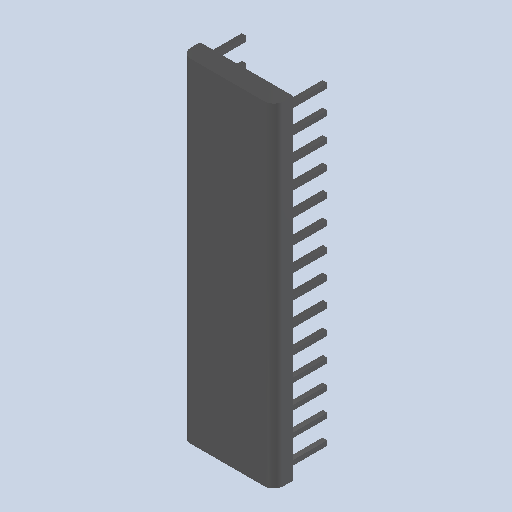
# Autodesk Inventor part: ATMEGA328P-PV
Saved by Autodesk Inventor 2022 (Build 260153000, 153)
## iProperties
Created: 2017-06-03
Part Number: ATMEGA328P-PV
Material: Rubber
Document SubType Name: Modeling
Designer: L.Đ.P
Density: 0.93 g/cm^3
Appearance: Rubber - Black - Version 1.1
Mass: 0.646794 g
Surface Area: 10.546 cm^2
Volume: 0.695478 cm^3
Author: L.Đ.P
Autodesk Inventor part; units mm, degrees
ref_plane "YZ Plane" through (0, 0, 0) normal (1, 0, 0) x (0, 1, 0)
ref_plane "XZ Plane" through (0, 0, 0) normal (0, 1, 0) x (-1, 0, 0)
ref_plane "XY Plane" through (0, 0, 0) normal (0, 0, 1) x (1, 0, 0)
sketch "Sketch1" plane through (0, 0, 0) normal (0, 0, 1) x (1, 0, 0)
  line L0 (0.625, 15.75) -> (0.625, 16.75) projected
  line L1 (0.625, 16.75) -> (-0.625, 16.75) projected
  line L2 (-0.625, 16.75) -> (-0.625, 18.25) projected
  line L3 (-0.625, 18.25) -> (0.625, 18.25) projected
  line L4 (0.625, 18.25) -> (0.625, 19.25) projected
  line L5 (0.625, 19.25) -> (-0.625, 19.25) projected
  line L6 (-0.625, 19.25) -> (-0.625, 20.75) projected
  line L7 (-0.625, 20.75) -> (0.625, 20.75) projected
  line L8 (0.625, 20.75) -> (0.625, 21.75) projected
  line L9 (0.625, 21.75) -> (-0.625, 21.75) projected
  line L10 (-0.625, 21.75) -> (-0.625, 23.25) projected
  line L11 (-0.625, 23.25) -> (0.625, 23.25) projected
  line L12 (0.625, 23.25) -> (0.625, 24.25) projected
  line L13 (0.625, 24.25) -> (-0.625, 24.25) projected
  line L14 (-0.625, 24.25) -> (-0.625, 25.75) projected
  line L15 (-0.625, 25.75) -> (0.625, 25.75) projected
  line L16 (0.625, 25.75) -> (0.625, 26.75) projected
  line L17 (0.625, 26.75) -> (-0.625, 26.75) projected
  line L18 (-0.625, 26.75) -> (-0.625, 28.25) projected
  line L19 (-0.625, 28.25) -> (0.625, 28.25) projected
  line L20 (0.625, 28.25) -> (0.625, 29.25) projected
  line L21 (0.625, 29.25) -> (-0.625, 29.25) projected
  line L22 (-0.625, 29.25) -> (-0.625, 30.75) projected
  line L23 (-0.625, 30.75) -> (0.625, 30.75) projected
  line L24 (0.625, 30.75) -> (0.625, 31.75) projected
  line L25 (0.625, 31.75) -> (-0.625, 31.75) projected
  line L26 (-0.625, 31.75) -> (-0.625, 33.25) projected
  line L27 (-0.625, 33.25) -> (0.625, 33.25) projected
  line L28 (0.625, 33.25) -> (0.625, 33.75) projected
  line L29 (0.625, 33.75) -> (-9.125, 33.75) projected
  line L30 (-9.125, 33.75) -> (-9.125, 33.25) projected
  line L31 (-9.125, 33.25) -> (-7.875, 33.25) projected
  line L32 (-7.875, 33.25) -> (-7.875, 31.75) projected
  line L33 (-7.875, 31.75) -> (-9.125, 31.75) projected
  line L34 (-9.125, 31.75) -> (-9.125, 30.75) projected
  line L35 (-9.125, 30.75) -> (-7.875, 30.75) projected
  line L36 (-7.875, 30.75) -> (-7.875, 29.25) projected
  line L37 (-7.875, 29.25) -> (-9.125, 29.25) projected
  line L38 (-9.125, 29.25) -> (-9.125, 28.25) projected
  line L39 (-9.125, 28.25) -> (-7.875, 28.25) projected
  line L40 (-7.875, 28.25) -> (-7.875, 26.75) projected
  line L41 (-7.875, 26.75) -> (-9.125, 26.75) projected
  line L42 (-9.125, 26.75) -> (-9.125, 25.75) projected
  line L43 (-9.125, 25.75) -> (-7.875, 25.75) projected
  line L44 (-7.875, 25.75) -> (-7.875, 24.25) projected
  line L45 (-7.875, 24.25) -> (-9.125, 24.25) projected
  line L46 (-9.125, 24.25) -> (-9.125, 23.25) projected
  line L47 (-9.125, 23.25) -> (-7.875, 23.25) projected
  line L48 (-7.875, 23.25) -> (-7.875, 21.75) projected
  line L49 (-7.875, 21.75) -> (-9.125, 21.75) projected
  line L50 (-9.125, 21.75) -> (-9.125, 20.75) projected
  line L51 (-9.125, 20.75) -> (-7.875, 20.75) projected
  line L52 (-7.875, 20.75) -> (-7.875, 19.25) projected
  line L53 (-7.875, 19.25) -> (-9.125, 19.25) projected
  line L54 (-9.125, 19.25) -> (-9.125, 18.25) projected
  line L55 (-9.125, 18.25) -> (-7.875, 18.25) projected
  line L56 (-7.875, 18.25) -> (-7.875, 16.75) projected
  line L57 (-7.875, 16.75) -> (-9.125, 16.75) projected
  line L58 (-9.125, 16.75) -> (-9.125, 15.75) projected
  line L59 (-9.125, 15.75) -> (-7.875, 15.75) projected
  line L60 (-7.875, 15.75) -> (-7.875, 14.25) projected
  line L61 (-7.875, 14.25) -> (-9.125, 14.25) projected
  line L62 (-9.125, 14.25) -> (-9.125, 13.25) projected
  line L63 (-9.125, 13.25) -> (-7.875, 13.25) projected
  line L64 (-7.875, 13.25) -> (-7.875, 11.75) projected
  line L65 (-7.875, 11.75) -> (-9.125, 11.75) projected
  line L66 (-9.125, 11.75) -> (-9.125, 10.75) projected
  line L67 (-9.125, 10.75) -> (-7.875, 10.75) projected
  line L68 (-7.875, 10.75) -> (-7.875, 9.25) projected
  line L69 (-7.875, 9.25) -> (-9.125, 9.25) projected
  line L70 (-9.125, 9.25) -> (-9.125, 8.25) projected
  line L71 (-9.125, 8.25) -> (-7.875, 8.25) projected
  line L72 (-7.875, 8.25) -> (-7.875, 6.75) projected
  line L73 (-7.875, 6.75) -> (-9.125, 6.75) projected
  line L74 (-9.125, 6.75) -> (-9.125, 5.75) projected
  line L75 (-9.125, 5.75) -> (-7.875, 5.75) projected
  line L76 (-7.875, 5.75) -> (-7.875, 4.25) projected
  line L77 (-7.875, 4.25) -> (-9.125, 4.25) projected
  line L78 (-9.125, 4.25) -> (-9.125, 3.25) projected
  line L79 (-9.125, 3.25) -> (-7.875, 3.25) projected
  line L80 (-7.875, 3.25) -> (-7.875, 1.75) projected
  line L81 (-7.875, 1.75) -> (-9.125, 1.75) projected
  line L82 (-9.125, 1.75) -> (-9.125, 0.75) projected
  line L83 (-9.125, 0.75) -> (-7.875, 0.75) projected
  line L84 (-7.875, 0.75) -> (-7.875, -0.75) projected
  line L85 (-7.875, -0.75) -> (-9.125, -0.75) projected
  line L86 (-9.125, -0.75) -> (-9.125, -1.25) projected
  line L87 (-9.125, -1.25) -> (0.625, -1.25) projected
  line L88 (0.625, -1.25) -> (0.625, -0.75) projected
  line L89 (0.625, -0.75) -> (-0.625, -0.75) projected
  line L90 (-0.625, -0.75) -> (-0.625, 0.75) projected
  line L91 (-0.625, 0.75) -> (0.625, 0.75) projected
  line L92 (0.625, 0.75) -> (0.625, 1.75) projected
  line L93 (0.625, 1.75) -> (-0.625, 1.75) projected
  line L94 (-0.625, 1.75) -> (-0.625, 3.25) projected
  line L95 (-0.625, 3.25) -> (0.625, 3.25) projected
  line L96 (0.625, 3.25) -> (0.625, 4.25) projected
  line L97 (0.625, 4.25) -> (-0.625, 4.25) projected
  line L98 (-0.625, 4.25) -> (-0.625, 5.75) projected
  line L99 (-0.625, 5.75) -> (0.625, 5.75) projected
  line L100 (0.625, 5.75) -> (0.625, 6.75) projected
  line L101 (0.625, 6.75) -> (-0.625, 6.75) projected
  line L102 (-0.625, 6.75) -> (-0.625, 8.25) projected
  line L103 (-0.625, 8.25) -> (0.625, 8.25) projected
  line L104 (0.625, 8.25) -> (0.625, 9.25) projected
  line L105 (0.625, 9.25) -> (-0.625, 9.25) projected
  line L106 (-0.625, 9.25) -> (-0.625, 10.75) projected
  line L107 (-0.625, 10.75) -> (0.625, 10.75) projected
  line L108 (0.625, 10.75) -> (0.625, 11.75) projected
  line L109 (0.625, 11.75) -> (-0.625, 11.75) projected
  line L110 (-0.625, 11.75) -> (-0.625, 13.25) projected
  line L111 (-0.625, 13.25) -> (0.625, 13.25) projected
  line L112 (0.625, 13.25) -> (0.625, 14.25) projected
  line L113 (0.625, 14.25) -> (-0.625, 14.25) projected
  line L114 (-0.625, 14.25) -> (-0.625, 15.75) projected
  line L115 (-0.625, 15.75) -> (0.625, 15.75) projected
  line L116 (-9.125, 33.75) -> (0.625, 33.75)
  line L117 (0.625, 33.75) -> (0.625, -1.25)
  line L118 (0.625, -1.25) -> (-9.125, -1.25)
  line L119 (-9.125, -1.25) -> (-9.125, 33.75)
  line L120 (0.25, -0.25) -> (-0.25, -0.25)
  line L121 (-0.25, -0.25) -> (-0.25, 0.25)
  line L122 (-0.25, 0.25) -> (0.25, 0.25)
  line L123 (0.25, 0.25) -> (0.25, -0.25)
  line L124 (0, 0) -> (0, -0.1911)
  line L125 (0, 0) -> (0.1004, 0)
  line L126 (-8.25, -0.25) -> (-8.75, -0.25)
  line L127 (-8.75, -0.25) -> (-8.75, 0.25)
  line L128 (-8.75, 0.25) -> (-8.25, 0.25)
  line L129 (-8.25, 0.25) -> (-8.25, -0.25)
  point P0 (0, 0.25)
  point P1 (0.25, 0)
  dimension "d2" = 0.5
  dimension "d3" = 0.5
  dimension "d4" = 0.5
  dimension "d5" = 0.5
  dimension "d6" = 0.375
  dimension "d7" = 0.5
  constraints: 28 end point, 7 parallel, 4 perpendicular, 3 horizontal, 2 midpoint, 2 point on line
  measures "d2" distance of L121.end L122.end
  measures "d3" distance of L120.end L121.end
  measures "d4" distance of L127.end L128.end
  measures "d5" distance of L126.end L127.end
  measures "d6" distance between parallel lines of L84 L129
  measures "d7" distance between parallel lines of L83 L128
extrude "Extrusion1" add sketch "Sketch1" along normal blind 2 contours L115 L114 L113 L112 L111 L110 L109 L108 L107 L106 L105 L104 L103 L102 L101 L100 L99 L98 L97 L96 L95 L94 L93 L92 L91 L90 L89 L88 L87 L86 L85 L84 L83 L82 L81 L80 L79 L78 L77 L76 L75 L74 L73 L72 L71 L70 L69 L68 L67 L66 L65 L64 L63 L62 L61 L60 L59 L58 L57 L56 L55 L54 L53 L52 L51 L50 L49 L48 L47 L46 L45 L44 L43 L42 L41 L40 L39 L38 L37 L36 L35 L34 L33 L32 L31 L30 L29 L28 L27 L26 L25 L24 L23 L22 L21 L20 L19 L18 L17 L16 L15 L14 L13 L12 L11 L10 L9 L8 L7 L6 L5 L4 L3 L2 L1 L0 | L117 L113 L114 L115 | L1 L2 L3 L117 | L117 L109 L110 L111 | L5 L6 L7 L117 | L117 L105 L106 L107 | L9 L10 L11 L117 | L117 L101 L102 L103 | L13 L14 L15 L117 | L117 L97 L98 L99 | L17 L18 L19 L117 | L117 L93 L94 L95 | L21 L22 L23 L117 | L117 L89 L90 L91 | L25 L26 L27 L117 | L119 L83 L84 L85 | L31 L32 L33 L119 | L119 L79 L80 L81 | L35 L36 L37 L119 | L119 L75 L76 L77 | L39 L40 L41 L119 | L119 L71 L72 L73 | L43 L44 L45 L119 | L119 L67 L68 L69 | L47 L48 L49 L119 | L119 L63 L64 L65 | L51 L52 L53 L119 | L119 L59 L60 L61 | L55 L56 L57 L119 | L120 L121 L122 L123 | L126 L127 L128 L129
extrude "Extrusion2" add sketch "Sketch1" against normal blind 4 contours L120 L121 L122 L123 | L126 L127 L128 L129
pattern_linear "Rectangular Pattern1" count 14 spacing 2.5 along (0, 1, 0) of "Extrusion2"
fillet "Fillet1" radius 1 2 edges at (0.625, 16.25, 2) (-9.125, 16.25, 2)
body "Solid1"
